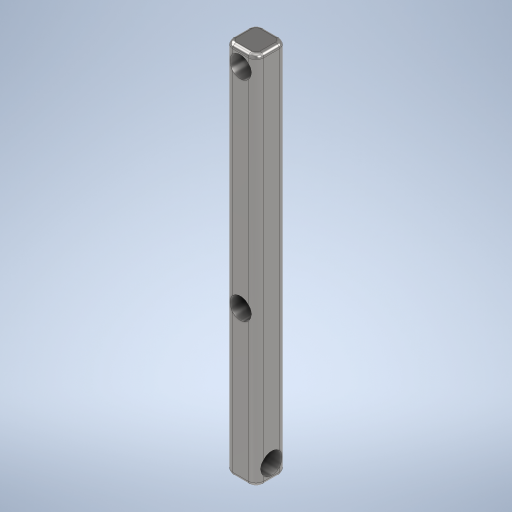
# Autodesk Inventor part: beam
Saved by Autodesk Inventor 2023 (Build 270158000, 158)
## iProperties
Created: 2022-09-27
Part Number: beam
Material: Stainless Steel
Document SubType Name: Modeling
Designer: aaron
Density: 8 g/cm^3
Appearance: Semi-Polished
Author: aaron
Autodesk Inventor part; units mm, degrees
ref_plane "YZ Plane" through (0, 0, 0) normal (1, 0, 0) x (0, 1, 0)
ref_plane "XZ Plane" through (0, 0, 0) normal (0, 1, 0) x (-1, 0, 0)
ref_plane "XY Plane" through (0, 0, 0) normal (0, 0, 1) x (1, 0, 0)
sketch "Sketch1" plane through (0, 0, 0) normal (0, 1, 0) x (-1, 0, 0)
  line L0 (-3.175, -3.175) -> (3.175, -3.175)
  line L1 (3.175, -3.175) -> (3.175, 3.175)
  line L2 (3.175, 3.175) -> (-3.175, 3.175)
  line L3 (-3.175, 3.175) -> (-3.175, -3.175)
  line L4 (-3.175, -3.175) -> (3.175, 3.175) construction
  line L5 (3.175, -3.175) -> (-3.175, 3.175) construction
  point P0 (0, 0)
  dimension "d0" = 6.35
  dimension "d1" = 6.35
  constraints: 12 end point, 2 midpoint, 2 parallel, 1 horizontal, 1 perpendicular
  measures "d0" distance of L2.end L1.end
  measures "d1" distance of L1.end L0.end
extrude "Extrusion1" add sketch "Sketch1" along normal blind 76.2
sketch "Sketch2" plane through (3.175, 0, 3.175) normal (1, 0, 0) x (0, 0, -1)
  circle A0 centre (3.175, 3.175) radius 2.159
  line L0 (0, 0) -> (6.35, 0) projected
  point P0 (3.175, 0)
  dimension "d4" = 4.318
  dimension "d5" = 3.175
  constraints: 1 centre point
  measures "d4" diameter of A0
  measures "d5" distance from line of L0 A0.centre
extrude "Extrusion2" cut sketch "Sketch2" against normal blind 76.2
fillet "Fillet1" radius 1.5875 4 edges at (3.175, 38.1, -3.175) (-3.175, 38.1, -3.175) (3.175, 38.1, 3.175) (-3.175, 38.1, 3.175)
fillet "Fillet2" radius 0.7937 16 edges at (2.71, 0, 2.71) (3.175, 0, 0) (2.71, 0, -2.71) (0, 0, -3.175) (-2.71, 0, -2.71) (-3.175, 0, 0) (-2.71, 0, 2.71) (0, 0, 3.175) (2.71, 76.2, 2.71) (3.175, 76.2, 0) (2.71, 76.2, -2.71) (0, 76.2, -3.175) (-2.71, 76.2, -2.71) (-3.175, 76.2, 0) (-2.71, 76.2, 2.71) (0, 76.2, 3.175)
sketch "Sketch3" plane through (-1.5875, 75.4062, 3.175) normal (0, 0, 1) x (1, 0, 0)
  circle A0 centre (1.5875, -44.9263) radius 2.159
  line L0 (0, -75.4062) -> (3.175, -75.4062) projected
  point P0 (1.5875, -75.4062)
  dimension "d10" = 4.318
  dimension "d11" = 30.48
  constraints: 1 centre point
  measures "d10" diameter of A0
  measures "d11" distance from line of L0 A0.centre
extrude "Extrusion3" cut sketch "Sketch3" against normal blind 76.2
sketch "Sketch4" plane through (-1.5875, 75.4062, 3.175) normal (0, 0, 1) x (1, 0, 0)
  circle A0 centre (1.5875, -2.3813) radius 2.159
  line L0 (3.175, 0.7937) -> (0, 0.7937) projected
  point P0 (1.5875, -75.4062)
  dimension "d14" = 4.318
  dimension "d15" = 3.175
  constraints: 1 centre point
  measures "d14" diameter of A0
  measures "d15" distance from line of L0 A0.centre
extrude "Extrusion4" cut sketch "Sketch4" against normal blind 76.2
body "Solid1"
